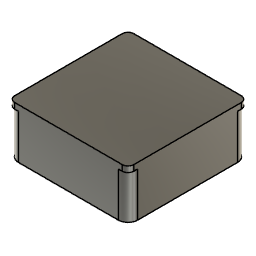
Box v1 (1) (Autodesk Fusion 360 design; units mm, degrees)
Autodesk Fusion 360 part; units mm, degrees
sketch "Sketch1" plane through (0, 0, 0) normal (0, 0, 1) x (1, 0, 0)
  line L0 (155, 155) -> (-155, 155)
  line L1 (-155, 155) -> (-155, -155)
  line L2 (-155, -155) -> (155, -155)
  line L3 (155, -155) -> (155, 155)
  line L4 (155, 155) -> (-155, -155) construction
  line L5 (-155, 155) -> (155, -155) construction
  dimension "d1" = 310
  dimension "d2" = 310
  constraint horizontal L0
  constraint perpendicular L0 L1
  constraint parallel L0 L2
  constraint parallel L1 L3
  constraint coincident L4 origin
  constraint coincident L5 origin
  measures "d1" distance of L1.end L2.end
  measures "d2" distance of L0.end L1.end
extrude "Extrude1" add sketch "Sketch1" along normal blind 115
shell "Shell1" thickness 10 removed faces 1 at (-51.6667, 51.6667, 115)
fillet "Fillet1" radius 25 4 edges at (-155, -155, 57.5) (155, -155, 57.5) (-155, 155, 57.5) (155, 155, 57.5)
ref_plane "WorkPlane1" through (0, 0, 115) normal (0, 0, 1) x (1, 0, 0)
sketch "Sketch2" plane through (0, 0, 115) normal (0, 0, 1) x (1, 0, 0)
  line L0 (155, 155) -> (-155, 155)
  line L1 (-155, 155) -> (-155, -155)
  line L2 (-155, -155) -> (155, -155)
  line L3 (155, -155) -> (155, 155)
  line L4 (155, 155) -> (-155, -155) construction
  line L5 (-155, 155) -> (155, -155) construction
  line L6 (-145, 145) -> (145, 145)
  line L7 (145, 145) -> (145, -145)
  line L8 (145, -145) -> (-145, -145)
  line L9 (-145, -145) -> (-145, 145)
  line L10 (-145, 145) -> (145, -145) construction
  line L11 (145, 145) -> (-145, -145) construction
  dimension "d9" = 310
  dimension "d10" = 310
  dimension "d11" = 290
  dimension "d12" = 290
  constraint horizontal L0
  constraint perpendicular L0 L1
  constraint parallel L0 L2
  constraint parallel L1 L3
  constraint coincident L4 origin
  constraint coincident L5 origin
  constraint horizontal L6
  constraint perpendicular L6 L7
  constraint parallel L6 L8
  constraint parallel L7 L9
  constraint coincident L10 origin
  constraint coincident L11 origin
  measures "d9" distance of L1.end L2.end
  measures "d10" distance of L0.end L1.end
  measures "d11" distance of L7.end L8.end
  measures "d12" distance of L6.end L7.end
extrude "Extrude2" add sketch "Sketch2" against normal blind 15 contours L6 L7 L8 L9
extrude "Extrude3" add sketch "Sketch2" along normal blind 15 contours L0 L1 L2 L3 | L6 L7 L8 L9
fillet "Fillet2" radius 15 4 edges at (-155, 155, 122.5) (-155, -155, 122.5) (155, -155, 122.5) (155, 155, 122.5)
